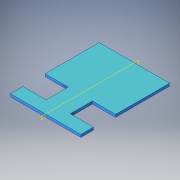
# Autodesk Inventor part: RhinoBottomFloorPlate02
Saved by Autodesk Inventor 2016 SP1 (Build 200210100, 210)
## iProperties
Created: 2015-12-30
Part Number: RhinoBottomFloorPlate02
Material: Wood (Birch)
Document SubType Name: Modeling
Designer: steele
Density: 0.55 g/cm^3
Appearance: Cyan
Mass: 3217.6 g
Surface Area: 6616.12 cm^2
Volume: 5850.18 cm^3
Author: steele
Autodesk Inventor part; units mm, degrees
ref_plane "XZ Plane" through (0, 0, 0) normal (0, 1, 0) x (-1, 0, 0)
ref_plane "XY Plane" through (0, 0, 0) normal (0, 0, 1) x (1, 0, 0)
sketch "Sketch1" plane through (0, 0, 0) normal (0, 1, 0) x (-1, 0, 0)
  line L0 (-231.775, 292.1) -> (-231.775, -292.1)
  line L1 (-231.775, -292.1) -> (231.775, -292.1)
  line L2 (231.775, -292.1) -> (231.775, 292.1)
  line L3 (231.775, 292.1) -> (-231.775, 292.1)
  line L4 (-231.775, 292.1) -> (231.775, -292.1) construction
  line L5 (-231.775, -292.1) -> (231.775, 292.1) construction
  point P0 (0, 0)
  dimension "baseLength" = 584.2
  dimension "baseWidth" = 463.55
  constraints: 12 end point, 2 midpoint, 2 parallel, 1 perpendicular, 1 vertical
  measures "baseLength" distance of L0.start L0.end
  measures "baseWidth" distance of L2.end L0.start
extrude "Extrusion1" add sketch "Sketch1" along normal blind 17.78
sketch "Sketch2" plane through (0, 0, 0) normal (0, -1, 0) x (1, 0, 0)
  line L0 (231.775, 292.1) -> (231.775, -292.1) projected
  line L1 (231.775, 209.55) -> (79.375, 209.55)
  line L2 (79.375, 209.55) -> (79.375, 63.5)
  line L3 (79.375, 63.5) -> (231.775, 63.5)
  line L4 (231.775, 63.5) -> (231.775, 209.55)
  line L5 (-231.775, 292.1) -> (231.775, 292.1) projected
  point P0 (0, 0)
  dimension "backToEndOfGearBox" = 82.55
  dimension "backToFrontOfGearBox" = 228.6
  dimension "wdithForGearBox" = 152.4
  constraints: 8 end point, 2 perpendicular, 2 point on line, 1 collinear, 1 horizontal
  measures "backToEndOfGearBox" distance between parallel lines of L1 L5
  measures "backToFrontOfGearBox" distance between parallel lines of L3 L5
  measures "wdithForGearBox" distance between parallel lines of L2 L0
extrude "Extrusion2" cut sketch "Sketch2" against normal through all
mirror "Mirror1" about plane through (0, 0, 0) normal (1, 0, 0) of "Extrusion2"
equation "\"spaceingAlongSides\" = 3.175"
equation "\"distanceFromBackForEndBolt\" = 38.1"
equation "\"spacingForBolt\" = 25.4"
equation "\"widthOfSpacingForBolt\" = 12.7"
equation "\"lengthOfSpacingForBolt\" = 25.4"
body "Solid1"
